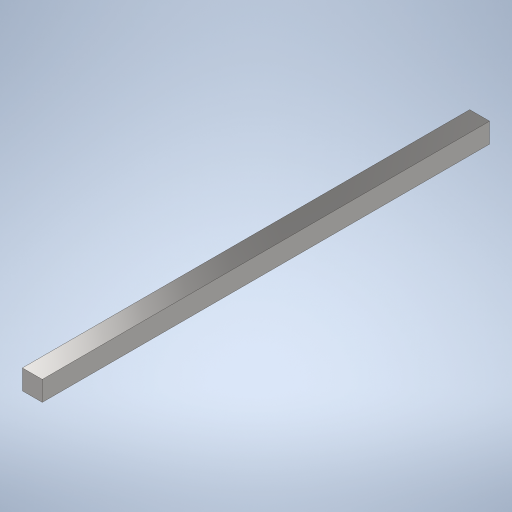
# Autodesk Inventor part: IC_pin
Saved by Autodesk Inventor 2023.1 (Build 271208000, 208)
## iProperties
Created: 2022-12-07
Part Number: IC_pin
Material: Stainless Steel
Document SubType Name: Modeling
Designer: mnelyubo
Density: 8 g/cm^3
Appearance: Semi-Polished
Author: mnelyubo
Autodesk Inventor part; units mm, degrees
ref_plane "YZ Plane" through (0, 0, 0) normal (1, 0, 0) x (0, 1, 0)
ref_plane "XZ Plane" through (0, 0, 0) normal (0, 1, 0) x (-1, 0, 0)
ref_plane "XY Plane" through (0, 0, 0) normal (0, 0, 1) x (1, 0, 0)
sketch "Sketch1" plane through (0, 0, 0) normal (0, 0, 1) x (1, 0, 0)
  line L0 (0, 0) -> (0.508, 0)
  line L1 (0.508, 0) -> (0.508, 0.508)
  line L2 (0.508, 0.508) -> (0, 0.508)
  line L3 (0, 0.508) -> (0, 0)
  dimension "d0" = 0.508
  dimension "d1" = 0.508
  constraints: 8 end point, 2 parallel, 1 horizontal, 1 perpendicular
  measures "d0" distance of L2.end L1.end
  measures "d1" distance of L1.end L0.end
extrude "Extrusion1" add sketch "Sketch1" along normal blind 11.43
body "Solid1"
